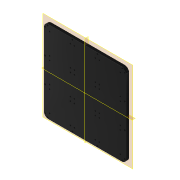
# Autodesk Inventor part: 30_XYTable_Aliexpress_Baseplate_aluminium_CNC
Saved by Autodesk Inventor 2022 (Build 260153000, 153)
## iProperties
Created: 2022-11-23
Part Number: 30_XYTable_Aliexpress_Baseplate_aluminium_CNC
Material: Generisch
Document SubType Name: Modeling
Designer: diederichbenedict
Density: 1 g/cm^3
Appearance: Glatt - Schwarz
Author: diederichbenedict
Autodesk Inventor part; units mm, degrees
ref_plane "YZ Plane" through (0, 0, 0) normal (1, 0, 0) x (0, 1, 0)
ref_plane "XZ Plane" through (0, 0, 0) normal (0, 1, 0) x (-1, 0, 0)
ref_plane "XY Plane" through (0, 0, 0) normal (0, 0, 1) x (1, 0, 0)
ref_plane "Arbeitsebene1" through (0, 0, 0) normal (0, 0, 1) x (1, 0, 0)
sketch "Skizze1" plane through (0, 0, 0) normal (0, 0, 1) x (1, 0, 0)
  arc A0 (22.6274, 8) -> (22.6274, -8) centre (0, 0) ccw
  line L0 (-73.5, 82.5) -> (73.5, 82.5)
  line L1 (82.5, 73.5) -> (82.5, -73.5)
  line L2 (73.5, -82.5) -> (-73.5, -82.5)
  line L3 (-82.5, -73.5) -> (-82.5, 73.5)
  line L4 (-82.5, 82.5) -> (82.5, -82.5) construction
  line L5 (82.5, 82.5) -> (-82.5, -82.5) construction
  arc A1 (73.5, -82.5) -> (82.5, -73.5) centre (73.5, -73.5) ccw
  arc A2 (-82.5, -73.5) -> (-73.5, -82.5) centre (-73.5, -73.5) ccw
  arc A3 (-73.5, 82.5) -> (-82.5, 73.5) centre (-73.5, 73.5) ccw
  arc A4 (82.5, 73.5) -> (73.5, 82.5) centre (73.5, 73.5) ccw
  arc A5 (77.5, -82.5) -> (82.5, -77.5) centre (77.5, -77.5) ccw construction
  arc A6 (73.5, -82.5) -> (82.5, -73.5) centre (73.5, -73.5) ccw construction
  dimension "d41" = 165
  dimension "d42" = 165
  dimension "d43" = 9
  constraints: 14 point on circle, 12 end point, 8 point on line, 8 tangent, 7 centre point, 3 equal radius, 2 midpoint, 2 parallel, 1 horizontal, 1 perpendicular, 12 other
  measures "d41" distance of L4.end L5.end
  measures "d42" distance of L5.start L4.end
  measures "d43" radius of A1
extrude "Extrusion1" add sketch "Skizze1" along normal blind 6
sketch "Skizze2" plane through (0, 0, 6) normal (0, 0, 1) x (1, 0, 0)
  line L0 (-73.5, -82.5) -> (73.5, -82.5) projected
  arc A0 (82.5, -73.5) -> (73.5, -82.5) centre (73.5, -73.5) ccw projected
  line L1 (82.5, -73.5) -> (82.5, 73.5) projected
  arc A1 (73.5, 82.5) -> (82.5, 73.5) centre (73.5, 73.5) ccw projected
  line L2 (73.5, 82.5) -> (-73.5, 82.5) projected
  arc A2 (-82.5, 73.5) -> (-73.5, 82.5) centre (-73.5, 73.5) ccw projected
  line L3 (-82.5, 73.5) -> (-82.5, -73.5) projected
  arc A3 (-73.5, -82.5) -> (-82.5, -73.5) centre (-73.5, -73.5) ccw projected
  circle A4 centre (0, 0) radius 82.5
  line L4 (21, -21) -> (-21, -21) construction
  line L5 (-21, -21) -> (-21, 21) construction
  line L6 (-21, 21) -> (21, 21) construction
  line L7 (21, 21) -> (21, -21) construction
  line L8 (21, -21) -> (-21, 21) construction
  line L9 (-21, -21) -> (21, 21) construction
  point P0 (50.2, -0.2)
  point P1 (-49.9, 49.65)
  point P2 (50.2, 49.65)
  dimension "d47" = 42
  dimension "d48" = 42
  constraints: 12 end point, 3 tangent, 2 midpoint, 2 parallel, 1 centre point, 1 horizontal, 1 perpendicular
  measures "d47" distance of L5.end L6.end
  measures "d48" distance of L4.end L5.end
hole "Bohrung1" at (21, 21, 6) at (21, -21, 6) at (-21, -21, 6) at (-21, 21, 6) direction (0, 0, -1) diameter 2.9 end through all
sketch "Skizze3" plane through (0, 0, 0) normal (0, 0, -1) x (-1, 0, 0)
  circle A0 centre (-50.2, -0.2) radius 2.4 projected
  circle A1 centre (-50.2, 49.65) radius 2.4 projected
  circle A2 centre (49.9, 49.65) radius 2.4 projected
  circle A3 centre (49.9, 49.65) radius 6.5
  circle A4 centre (49.9, -0.1) radius 2.4 projected
  circle A5 centre (49.9, -0.1) radius 6.5
  circle A6 centre (49.9, -50.1) radius 2.4 projected
  circle A7 centre (49.9, -50.1) radius 6.5
  circle A8 centre (-0.1, -50.1) radius 2.4 projected
  circle A9 centre (-0.1, -50.1) radius 6.5
  circle A10 centre (0, 0) radius 6.5
  circle A11 centre (-0.15, 49.65) radius 2.4 projected
  circle A12 centre (-0.15, 49.65) radius 6.5
  circle A13 centre (-50.2, 49.65) radius 2.4 projected
  circle A14 centre (-50.2, 49.65) radius 6.5
  circle A15 centre (-50.2, -0.2) radius 2.4 projected
  circle A16 centre (-50.2, -0.2) radius 6.5
  circle A17 centre (-50.05, -50.05) radius 6.5
  dimension "d10" = 13
  dimension "d11" = 13
  dimension "d12" = 13
  dimension "d13" = 13
  dimension "d14" = 13
  dimension "d15" = 13
  dimension "d16" = 13
  dimension "d17" = 13
  dimension "d18" = 13
  constraints: 9 centre point, 7 coincident
  measures "d10" diameter of A3
  measures "d11" diameter of A5
  measures "d12" diameter of A7
  measures "d13" diameter of A9
  measures "d14" diameter of A10
  measures "d15" diameter of A12
  measures "d16" diameter of A14
  measures "d17" diameter of A16
  measures "d18" diameter of A17
hole "Bohrung2" [suppressed]
sketch "Skizze4" plane through (0, 0, 0) normal (0, 0, -1) x (-1, 0, 0)
  circle A0 centre (80, -25) radius 1.4
  circle A1 centre (80, 25) radius 1.4
  circle A2 centre (80, -25) radius 1.4
  circle A3 centre (80, -75) radius 1.4
  circle A4 centre (75, -80) radius 1.4
  circle A5 centre (25, -80) radius 1.4
  circle A6 centre (-25, -80) radius 1.4
  circle A7 centre (80, 25) radius 1.4
  circle A8 centre (25, -80) radius 1.4
  circle A9 centre (-25, -80) radius 1.4
  circle A10 centre (-75, -80) radius 1.4
  point P0 (0, 0)
  point P1 (79.2375, -30)
  point P2 (79.2375, 30)
  point P3 (79.2375, 60)
  point P4 (79.2375, -60)
  constraints: 11 centre point, 26 other
hole "Bohrung3" at (-75, -80, 0) at (-25, -80, 0) at (25, -80, 0) at (75, -80, 0) direction (0, 0, 1) diameter 3.5 end through all
ref_plane "Arbeitsebene2" through (0, -73.5, 0) normal (1, 0, 0) x (0, 0, -1)
ref_plane "Arbeitsebene3" through (-73.5, 0, 0) normal (0, 1, 0) x (1, 0, 0)
pattern_circular "Runde Anordnung2" count 4 over 360 about axis through (0, 0, 0) along (0, 0, -1) of "Bohrung3"
pattern_linear "Rechteckige Anordnung2" count 3 spacing 50 along (-1, 0, 0) count 3 spacing 50 along (0, -1, 0) of "Bohrung1" first direction both ways yes second direction both ways yes
chamfer "Fase1" distance 0.4 angle 45 8 edges at (79.864, 79.864, 6) (82.5, 0, 6) (79.864, -79.864, 6) (0, -82.5, 6) (-79.864, -79.864, 6) (-82.5, 0, 6) (-79.864, 79.864, 6) (0, 82.5, 6)
sketch "Skizze5" plane through (0, 0, 0) normal (0, 0, -1) x (-1, 0, 0)
  circle A0 centre (71, -71) radius 1.45 projected
  circle A1 centre (71, -29) radius 1.45 projected
  circle A2 centre (29, -71) radius 1.45 projected
  circle A3 centre (29, -29) radius 1.45 projected
  circle A4 centre (21, -71) radius 1.45 projected
  circle A5 centre (21, -29) radius 1.45 projected
  circle A6 centre (-21, -71) radius 1.45 projected
  circle A7 centre (-21, -29) radius 1.45 projected
  circle A8 centre (-29, -71) radius 1.45 projected
  circle A9 centre (-29, -29) radius 1.45 projected
  circle A10 centre (-71, -71) radius 1.45 projected
  circle A11 centre (-71, -29) radius 1.45 projected
  circle A12 centre (71, -21) radius 1.45 projected
  circle A13 centre (71, 21) radius 1.45 projected
  circle A14 centre (29, -21) radius 1.45 projected
  circle A15 centre (29, 21) radius 1.45 projected
  circle A16 centre (-29, -21) radius 1.45 projected
  circle A17 centre (-29, 21) radius 1.45 projected
  circle A18 centre (-71, -21) radius 1.45 projected
  circle A19 centre (-71, 21) radius 1.45 projected
  circle A20 centre (71, 29) radius 1.45 projected
  circle A21 centre (71, 71) radius 1.45 projected
  circle A22 centre (29, 29) radius 1.45 projected
  circle A23 centre (29, 71) radius 1.45 projected
  circle A24 centre (21, 29) radius 1.45 projected
  circle A25 centre (21, 71) radius 1.45 projected
  circle A26 centre (-21, 29) radius 1.45 projected
  circle A27 centre (-21, 71) radius 1.45 projected
  circle A28 centre (-29, 29) radius 1.45 projected
  circle A29 centre (-29, 71) radius 1.45 projected
  circle A30 centre (-71, 29) radius 1.45 projected
  circle A31 centre (-71, 71) radius 1.45 projected
  circle A32 centre (-80, 25) radius 1.75 projected
  circle A33 centre (-80, 75) radius 1.75 projected
  circle A34 centre (-80, -25) radius 1.75 projected
  circle A35 centre (-80, -75) radius 1.75 projected
  circle A36 centre (25, 80) radius 1.75 projected
  circle A37 centre (75, 80) radius 1.75 projected
  circle A38 centre (-25, 80) radius 1.75 projected
  circle A39 centre (-75, 80) radius 1.75 projected
  circle A40 centre (80, -25) radius 1.75 projected
  circle A41 centre (80, -75) radius 1.75 projected
  circle A42 centre (80, 25) radius 1.75 projected
  circle A43 centre (80, 75) radius 1.75 projected
  circle A44 centre (-25, -80) radius 1.75 projected
  circle A45 centre (75, -80) radius 1.75 projected
  circle A46 centre (25, -80) radius 1.75 projected
  circle A47 centre (-75, -80) radius 1.75 projected
  circle A48 centre (21, -21) radius 1.45 projected
  circle A49 centre (-21, 21) radius 1.45 projected
  circle A50 centre (-21, -21) radius 1.45 projected
  circle A51 centre (21, 21) radius 1.45 projected
  line L0 (73.5, -82.5) -> (-73.5, -82.5) projected
  arc A52 (73.5, -82.5) -> (82.5, -73.5) centre (73.5, -73.5) ccw projected
  line L1 (82.5, 73.5) -> (82.5, -73.5) projected
  arc A53 (82.5, 73.5) -> (73.5, 82.5) centre (73.5, 73.5) ccw projected
  line L2 (-73.5, 82.5) -> (73.5, 82.5) projected
  arc A54 (-73.5, 82.5) -> (-82.5, 73.5) centre (-73.5, 73.5) ccw projected
  line L3 (-82.5, -73.5) -> (-82.5, 73.5) projected
  arc A55 (-82.5, -73.5) -> (-73.5, -82.5) centre (-73.5, -73.5) ccw projected
  line L4 (-15.5, -17.5) -> (15.5, -17.5)
  line L5 (17.5, -15.5) -> (17.5, 15.5)
  line L6 (15.5, 17.5) -> (-15.5, 17.5)
  line L7 (-17.5, 15.5) -> (-17.5, -15.5)
  line L8 (-17.5, -17.5) -> (17.5, 17.5) construction
  line L9 (17.5, -17.5) -> (-17.5, 17.5) construction
  arc A56 (17.5, 15.5) -> (15.5, 17.5) centre (15.5, 15.5) ccw
  arc A57 (15.5, -17.5) -> (17.5, -15.5) centre (15.5, -15.5) ccw
  arc A58 (-17.5, -15.5) -> (-15.5, -17.5) centre (-15.5, -15.5) ccw
  arc A59 (-15.5, 17.5) -> (-17.5, 15.5) centre (-15.5, 15.5) ccw
  point P0 (0, 0)
  dimension "d58" = 35
  dimension "d59" = 35
  dimension "d60" = 2
  constraints: 12 end point, 8 point on circle, 8 point on line, 8 tangent, 4 centre point, 3 equal radius, 2 midpoint, 2 parallel, 1 horizontal, 1 perpendicular
  measures "d58" distance of L9.end L8.end
  measures "d59" distance of L8.end L9.start
  measures "d60" radius of A56
extrude "Extrusion3" cut sketch "Skizze5" against normal blind 5 contours A58 L7 A59 L6 A56 L5 A57 L4
pattern_linear "Rechteckige Anordnung3" count 3 spacing 50 along (0, 1, 0) count 3 spacing 50 along (1, 0, 0) of "Extrusion3" first direction both ways yes second direction both ways yes
